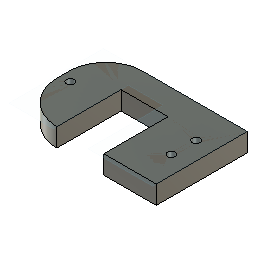
Motor Base V6 (Autodesk Fusion 360 design; units mm, degrees)
part number: Configuration 1
Autodesk Fusion 360 part; units mm, degrees
sketch "Sketch1" plane through (0, 0, 0) normal (0, 0, 1) x (1, 0, 0)
sketch "Sketch2" plane through (0, 0, 0) normal (0, 0, 1) x (1, 0, 0)
  line L0 (-65, -50) -> (51.4526, -50)
  line L1 (51.4526, -50) -> (51.4526, 26.6833)
  line L2 (51.4526, 26.6833) -> (-65, 26.6833)
  line L3 (-65, 26.6833) -> (-65, -50)
  constraint horizontal L0
  constraint vertical L1
  constraint horizontal L2
  constraint vertical L3
extrude "Extrude1" add sketch "Sketch2" along normal blind 15
sketch "Sketch3" plane through (0, 0, 15) normal (0, 0, 1) x (-1, 0, 0)
  line L0 (65, -26.6833) -> (65, 50)
  line L1 (65, 50) -> (-51.4526, 50)
  line L2 (-51.4526, 50) -> (-51.4526, -26.6833)
  line L3 (-51.4526, -26.6833) -> (65, -26.6833)
  line L4 (42.1958, 9.8978) -> (27.1958, 9.8978)
  line L5 (-16.8436, 9.8978) -> (3.1564, 9.8978)
  line L6 (1, 15) -> (1, -10.9397)
  line L7 (1, -10.9397) -> (28.9988, -10.9397)
  line L8 (28.9988, -10.9397) -> (28.9988, 52.9619)
  line L9 (28.9988, 52.9619) -> (1, 52.9619)
  line L10 (1, 52.9619) -> (1, -10.9397)
  dimension "d3" = 15
  dimension "d4" = 20
  constraint horizontal L4
  constraint horizontal L5
  constraint vertical L6
  constraint horizontal L7
  constraint vertical L8
  constraint horizontal L9
  constraint vertical L10
  measures "d3" distance of L4.start L4.end
  measures "d4" distance of L5.start L5.end
extrude "Extrude2" cut sketch "Sketch3" against normal blind 25 contours L1 L6 L7 L8 L10
sketch "Sketch4" plane through (0, 0, 15) normal (0, 0, 1) x (-1, 0, 0)
  line L0 (1, -10.9397) -> (1, 50)
  line L1 (1, 50) -> (-51.4526, 50)
  line L2 (-51.4526, 50) -> (-51.4526, -26.6833)
  line L3 (-51.4526, -26.6833) -> (65, -26.6833)
  line L4 (65, -26.6833) -> (65, 50)
  line L5 (65, 50) -> (28.9988, 50)
  line L6 (28.9988, 50) -> (28.9988, -10.9397)
  line L7 (28.9988, -10.9397) -> (1, -10.9397)
extrude "Extrude3" cut 1 faces at (-1, -29.6868, 10) along direction (1, 0, 0) blind 10
sketch "Sketch5" plane through (0, 0, 15) normal (0, 0, 1) x (-1, 0, 0)
extrude "Extrude4" add 1 faces at (-3.6663, 10.9397, 10) along direction (0, -1, 0) blind 6
extrude "Extrude5" cut 1 faces at (-65, 1.1222, 5) along direction (1, 0, 0) blind 2
extrude "Extrude6" cut 1 faces at (23.1509, -50, 5) along direction (0, 1, 0) blind 3
extrude "Extrude7" cut 1 faces at (-51.6663, -50, 5) along direction (0, 1, 0) blind 3
fillet "Fillet1" radius 35 1 edges at (-63, -47, 7.5)
fillet "Fillet2" radius 30 1 edges at (-63, 26.6833, 7.5)
hole "Hole1" at (-55.0963, -10.0219, 0) direction (0, 0, 1) diameter 6.3 depth 15 tip angle 118
hole "Hole2" at (36.7832, -20.0408, 0) direction (0, 0, 1) diameter 6.3 depth 15 tip angle 118
hole "Hole3" at (36.9862, -0.2374, 0) direction (0, 0, 1) diameter 6.3 depth 15 tip angle 118
